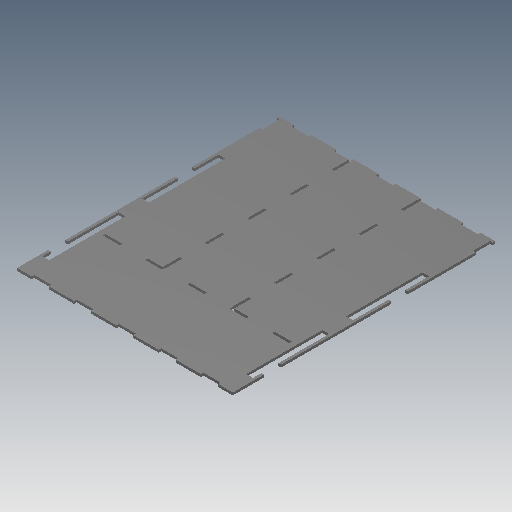
# Autodesk Inventor part: base
Saved by Autodesk Inventor 2020 (Build 240168000, 168)
## iProperties
Created: 2021-09-21
Part Number: base
Material: Generic
Document SubType Name: Modeling
Designer: pablo
Density: 1 g/cm^3
Appearance: Smooth - Black
Mass: 365.55 g
Surface Area: 1587.23 cm^2
Volume: 365.55 cm^3
Author: pablo
Autodesk Inventor part; units mm, degrees
ref_plane "YZ Plane" through (0, 0, 0) normal (1, 0, 0) x (0, 1, 0)
ref_plane "XZ Plane" through (0, 0, 0) normal (0, 1, 0) x (-1, 0, 0)
ref_plane "XY Plane" through (0, 0, 0) normal (0, 0, 1) x (1, 0, 0)
sketch "Sketch1" plane through (0, 0, 0) normal (0, 1, 0) x (-1, 0, 0)
  line L0 (127.5, -155) -> (-127.5, -155)
  line L1 (-127.5, -155) -> (-127.5, 155)
  line L2 (-127.5, 155) -> (127.5, 155)
  line L3 (127.5, 155) -> (127.5, -155)
  line L4 (127.5, -155) -> (-127.5, 155) construction
  line L5 (-127.5, -155) -> (127.5, 155) construction
  point P0 (0, 0)
  dimension "d0" = 255
  dimension "d1" = 310
  constraints: 12 end point, 2 midpoint, 2 parallel, 1 horizontal, 1 perpendicular
  measures "d0" distance of L1.end L2.end
  measures "d1" distance of L0.end L1.end
extrude "base" add sketch "Sketch1" along normal blind 3
sketch "Sketch4" plane through (0, 3, 0) normal (0, 1, 0) x (1, 0, 0)
  line L0 (-42.333, 152) -> (-39.333, 152)
  line L1 (-39.333, 152) -> (-39.333, 132)
  line L2 (-39.333, 132) -> (-42.333, 132)
  line L3 (-42.333, 132) -> (-42.333, 152)
  line L4 (39.3337, 152) -> (42.3337, 152)
  line L5 (42.3337, 152) -> (42.3337, 132)
  line L6 (42.3337, 132) -> (39.3337, 132)
  line L7 (39.3337, 132) -> (39.3337, 152)
  line L8 (-42.333, 102) -> (-39.333, 102)
  line L9 (-39.333, 102) -> (-39.333, 82)
  line L10 (-39.333, 82) -> (-42.333, 82)
  line L11 (-42.333, 82) -> (-42.333, 102)
  line L12 (39.3337, 102) -> (42.3337, 102)
  line L13 (42.3337, 102) -> (42.3337, 82)
  line L14 (42.3337, 82) -> (39.3337, 82)
  line L15 (39.3337, 82) -> (39.3337, 102)
  line L16 (-42.333, 52) -> (-39.333, 52)
  line L17 (-39.333, 52) -> (-39.333, 32)
  line L18 (-39.333, 32) -> (-42.333, 32)
  line L19 (-42.333, 32) -> (-42.333, 52)
  line L20 (39.3337, 52) -> (42.3337, 52)
  line L21 (42.3337, 52) -> (42.3337, 32)
  line L22 (42.3337, 32) -> (39.3337, 32)
  line L23 (39.3337, 32) -> (39.3337, 52)
  line L24 (-42.333, 2) -> (-39.333, 2)
  line L25 (-39.333, 2) -> (-39.333, -18)
  line L26 (-39.333, -18) -> (-42.333, -18)
  line L27 (-42.333, -18) -> (-42.333, 2)
  line L28 (39.3337, 2) -> (42.3337, 2)
  line L29 (42.3337, 2) -> (42.3337, -18)
  line L30 (42.3337, -18) -> (39.3337, -18)
  line L31 (39.3337, -18) -> (39.3337, 2)
  line L32 (-42.333, -48) -> (-39.333, -48)
  line L33 (-39.333, -48) -> (-39.333, -68)
  line L34 (-39.333, -68) -> (-42.333, -68)
  line L35 (-42.333, -68) -> (-42.333, -48)
  line L36 (39.3337, -48) -> (42.3337, -48)
  line L37 (42.3337, -48) -> (42.3337, -68)
  line L38 (42.3337, -68) -> (39.3337, -68)
  line L39 (39.3337, -68) -> (39.3337, -48)
  line L40 (0, 2.9944) -> (0, 16.9632)
  line L41 (127.5, 155) -> (-127.5, 155) projected
  point P0 (0, 0)
  dimension "d23" = 3
  dimension "d24" = 20
  dimension "d28" = 81.6667
  dimension "d31" = 50
  dimension "d93" = 39.333
  dimension "d94" = 39.3337
  dimension "d95" = 3
  constraints: 82 end point, 2 collinear, 2 horizontal, 2 parallel, 2 vertical, 1 perpendicular, 70 other
  measures "d23" distance of L1.end L2.end
  measures "d24" distance of L0.end L1.end
  measures "d28" distance of L0.start L4.start
  measures "d31" distance of L0.start L8.start
  measures "d93" horizontal distance of point (0, 0) L1.end
  measures "d94" horizontal distance of L6.end point (0, 0)
  measures "d95" distance from line of L41 L0.start
extrude "Encaixe Central" cut sketch "Sketch4" against normal blind 5
sketch "Sketch5" plane through (0, 3, 0) normal (0, 1, 0) x (1, 0, 0)
  line L0 (-127.5, -155) -> (127.5, -155) projected
  line L1 (-110, -155) -> (-90, -155)
  line L2 (-90, -155) -> (-90, -152)
  line L3 (-90, -152) -> (-110, -152)
  line L4 (-110, -152) -> (-110, -155)
  line L5 (-60, -155) -> (-40, -155)
  line L6 (-40, -155) -> (-40, -152)
  line L7 (-40, -152) -> (-60, -152)
  line L8 (-60, -152) -> (-60, -155)
  line L9 (-10, -155) -> (10, -155)
  line L10 (10, -155) -> (10, -152)
  line L11 (10, -152) -> (-10, -152)
  line L12 (-10, -152) -> (-10, -155)
  line L13 (40, -155) -> (60, -155)
  line L14 (60, -155) -> (60, -152)
  line L15 (60, -152) -> (40, -152)
  line L16 (40, -152) -> (40, -155)
  line L17 (90, -155) -> (110, -155)
  line L18 (110, -155) -> (110, -152)
  line L19 (110, -152) -> (90, -152)
  line L20 (90, -152) -> (90, -155)
  line L21 (-110, 155) -> (-110, 152)
  line L22 (-90, 155) -> (-110, 155)
  line L23 (-110, 152) -> (-90, 152)
  line L24 (-90, 152) -> (-90, 155)
  line L25 (-60, 155) -> (-60, 152)
  line L26 (-40, 155) -> (-60, 155)
  line L27 (-40, 152) -> (-40, 155)
  line L28 (-10, 155) -> (-10, 152)
  line L29 (10, 155) -> (-10, 155)
  line L30 (10, 152) -> (10, 155)
  line L31 (-10, 152) -> (10, 152)
  line L32 (-60, 152) -> (-40, 152)
  line L33 (40, 155) -> (40, 152)
  line L34 (40, 152) -> (60, 152)
  line L35 (60, 155) -> (40, 155)
  line L36 (60, 152) -> (60, 155)
  line L37 (90, 155) -> (90, 152)
  line L38 (90, 152) -> (110, 152)
  line L39 (110, 155) -> (90, 155)
  line L40 (110, 152) -> (110, 155)
  point P0 (0, 0)
  dimension "d36" = 20
  dimension "d37" = 3
  dimension "d40" = 50
  dimension "d45" = 17.5
  dimension "d46" = 17.5
  dimension "d49" = 307
  constraints: 80 end point, 2 horizontal, 2 parallel, 1 collinear, 1 perpendicular, 1 point on line, 1 vertical, 71 other
  measures "d36" distance of L3.end L2.end
  measures "d37" distance of L2.end L1.end
  measures "d40" distance of L1.start L5.start
  measures "d45" distance of L0.start L1.start
  measures "d46" distance of L17.end L0.end
  measures "d49" distance of L1.start L21.end
extrude "Encaixes frontais" cut sketch "Sketch5" against normal blind 5
sketch "Sketch6" plane through (0, 3, 0) normal (0, 1, 0) x (1, 0, 0)
  line L0 (-110, -155) -> (-110, -152) projected
  line L1 (110, -152) -> (110, -155) projected
  line L2 (-39.333, -68) -> (-42.333, -68) projected
  line L3 (-110, -68) -> (-90, -68)
  line L4 (-90, -68) -> (-90, -71)
  line L5 (-90, -71) -> (-110, -71)
  line L6 (-110, -71) -> (-110, -68)
  line L7 (-60, -68) -> (-40, -68)
  line L8 (-40, -68) -> (-40, -71)
  line L9 (-40, -71) -> (-60, -71)
  line L10 (-60, -71) -> (-60, -68)
  line L11 (-10, -68) -> (10, -68)
  line L12 (10, -68) -> (10, -71)
  line L13 (10, -71) -> (-10, -71)
  line L14 (-10, -71) -> (-10, -68)
  line L15 (40, -68) -> (60, -68)
  line L16 (60, -68) -> (60, -71)
  line L17 (60, -71) -> (40, -71)
  line L18 (40, -71) -> (40, -68)
  line L19 (90, -68) -> (110, -68)
  line L20 (110, -68) -> (110, -71)
  line L21 (110, -71) -> (90, -71)
  line L22 (90, -71) -> (90, -68)
  line L23 (-110, 155) -> (-127.5, 155) projected
  line L24 (-127.5, 155) -> (-127.5, -155) projected
  line L25 (127.5, -155) -> (127.5, 155) projected
  point P0 (0, 0)
  point P1 (-40, -68)
  dimension "d56" = 20
  dimension "d57" = 3
  dimension "d60" = 50
  dimension "d96" = 223
  dimension "d97" = 17.5
  dimension "d98" = 17.5
  constraints: 40 end point, 2 horizontal, 2 parallel, 1 collinear, 1 perpendicular, 31 other
  measures "d56" distance of L4.end L5.end
  measures "d57" distance of L3.end L4.end
  measures "d60" distance of L3.start L7.start
  measures "d96" distance from line of L23 L3.start
  measures "d97" distance from line of L24 L5.end
  measures "d98" distance from line of L25 L20.end
extrude "Encaixe longitudinal" cut sketch "Sketch6" against normal blind 5
sketch "Sketch7" plane through (0, 3, 0) normal (0, 1, 0) x (1, 0, 0)
  line L0 (-127.5, -155) -> (-110, -155) projected
  line L1 (-90, -155) -> (-60, -155) projected
  line L2 (-116.5, -10) -> (-124.5, -10)
  line L3 (-124.5, -10) -> (-124.5, 80)
  line L4 (-124.5, 80) -> (-116.5, 80)
  line L5 (-116.5, 80) -> (-116.5, -10)
  line L6 (-116.5, -10) -> (-124.5, 80) construction
  line L7 (-124.5, -10) -> (-116.5, 80) construction
  line L8 (-127.5, 155) -> (-127.5, -155) projected
  line L9 (-124.5, -128) -> (-116.5, -128)
  line L10 (-116.5, -128) -> (-116.5, -38)
  line L11 (-116.5, -38) -> (-124.5, -38)
  line L12 (-124.5, -38) -> (-124.5, -128)
  line L13 (-124.5, -128) -> (-116.5, -38) construction
  line L14 (-116.5, -128) -> (-124.5, -38) construction
  line L15 (0, -20) -> (0, -40)
  line L16 (116.5, -10) -> (124.5, -10)
  line L17 (124.5, -10) -> (124.5, 80)
  line L18 (124.5, 80) -> (116.5, 80)
  line L19 (116.5, 80) -> (116.5, -10)
  line L20 (116.5, -10) -> (124.5, 80) construction
  line L21 (124.5, -10) -> (116.5, 80) construction
  line L22 (127.5, -20) -> (127.5, -50)
  line L23 (124.5, -128) -> (116.5, -128)
  line L24 (116.5, -128) -> (116.5, -38)
  line L25 (116.5, -38) -> (124.5, -38)
  line L26 (124.5, -38) -> (124.5, -128)
  line L27 (124.5, -128) -> (116.5, -38) construction
  line L28 (116.5, -128) -> (124.5, -38) construction
  point P0 (0, 0)
  point P1 (-120.5, 35)
  point P2 (-127.5, -20)
  point P3 (-127.5, -50)
  point P4 (-120.5, -83)
  point P5 (120.5, 35)
  point P6 (120.5, -83)
  point P7 (-127.5, 150)
  dimension "d67" = 8
  dimension "d68" = 90
  dimension "d69" = 3
  dimension "d71" = 8
  dimension "d72" = 90
  dimension "d78" = 3
  dimension "d79" = 27
  dimension "d80" = 145
  constraints: 52 end point, 12 symmetric about line, 8 midpoint, 4 parallel, 2 horizontal, 2 perpendicular, 1 vertical
  measures "d67" distance of L3.end L4.end
  measures "d68" distance of L2.end L3.end
  measures "d69" distance from line of L8 L2.end
  measures "d71" distance of L11.end L10.end
  measures "d72" distance of L10.end L9.end
  measures "d78" horizontal distance of L0.start L9.start
  measures "d79" vertical distance of L0.start L9.start
  measures "d80" vertical distance of L0.start L2.end
extrude "Trajeto dos cursores" cut sketch "Sketch7" against normal blind 5
sketch "Sketch8" plane through (0, 3, 0) normal (0, 1, 0) x (1, 0, 0)
  line L0 (-127.5, 155) -> (-127.5, -155) projected
  line L1 (-110, 155) -> (-127.5, 155) projected
  line L2 (-127.5, 152) -> (-124.5, 152)
  line L3 (-124.5, 152) -> (-124.5, 132)
  line L4 (-124.5, 132) -> (-127.5, 132)
  line L5 (-127.5, 132) -> (-127.5, 152)
  line L6 (-90, 152) -> (-110, 152) projected
  line L7 (-42.333, 152) -> (-60, 152) projected
  line L8 (-127.5, 102) -> (-124.5, 102)
  line L9 (-124.5, 102) -> (-124.5, 82)
  line L10 (-124.5, 82) -> (-127.5, 82)
  line L11 (-127.5, 82) -> (-127.5, 102)
  line L12 (-127.5, 52) -> (-124.5, 52)
  line L13 (-124.5, 52) -> (-124.5, 32)
  line L14 (-124.5, 32) -> (-127.5, 32)
  line L15 (-127.5, 32) -> (-127.5, 52)
  line L16 (-127.5, 2) -> (-124.5, 2)
  line L17 (-124.5, 2) -> (-124.5, -18)
  line L18 (-124.5, -18) -> (-127.5, -18)
  line L19 (-127.5, -18) -> (-127.5, 2)
  line L20 (-127.5, -48) -> (-124.5, -48)
  line L21 (-124.5, -48) -> (-124.5, -68)
  line L22 (-124.5, -68) -> (-127.5, -68)
  line L23 (-127.5, -68) -> (-127.5, -48)
  line L24 (-127.5, -98) -> (-124.5, -98)
  line L25 (-124.5, -98) -> (-124.5, -118)
  line L26 (-124.5, -118) -> (-127.5, -118)
  line L27 (-127.5, -118) -> (-127.5, -98)
  line L28 (0, 0) -> (0, 17.1399)
  line L29 (127.5, 152) -> (124.5, 152)
  line L30 (124.5, 152) -> (124.5, 132)
  line L31 (124.5, 132) -> (127.5, 132)
  line L32 (127.5, 132) -> (127.5, 152)
  line L33 (127.5, 102) -> (124.5, 102)
  line L34 (124.5, 102) -> (124.5, 82)
  line L35 (124.5, 82) -> (127.5, 82)
  line L36 (127.5, 82) -> (127.5, 102)
  line L37 (127.5, 52) -> (124.5, 52)
  line L38 (124.5, 52) -> (124.5, 32)
  line L39 (124.5, 32) -> (127.5, 32)
  line L40 (127.5, 32) -> (127.5, 52)
  line L41 (127.5, 2) -> (124.5, 2)
  line L42 (124.5, 2) -> (124.5, -18)
  line L43 (124.5, -18) -> (127.5, -18)
  line L44 (127.5, -18) -> (127.5, 2)
  line L45 (127.5, -48) -> (124.5, -48)
  line L46 (124.5, -48) -> (124.5, -68)
  line L47 (124.5, -68) -> (127.5, -68)
  line L48 (127.5, -68) -> (127.5, -48)
  line L49 (127.5, -98) -> (124.5, -98)
  line L50 (124.5, -98) -> (124.5, -118)
  line L51 (124.5, -118) -> (127.5, -118)
  line L52 (127.5, -118) -> (127.5, -98)
  point P0 (127.5, 155)
  dimension "d82" = 3
  dimension "d83" = 20
  dimension "d86" = 50
  constraints: 98 end point, 25 symmetric about line, 2 parallel, 2 vertical, 1 horizontal, 1 perpendicular, 1 point on line, 40 other
  measures "d82" distance of L3.end L4.end
  measures "d83" distance of L2.end L3.end
  measures "d86" distance of L2.start L8.start
extrude "Encaixes latereis" cut sketch "Sketch8" against normal blind 3 contours L2 L3 L4 L0 | L12 L13 L14 L0 | L24 L25 L26 L0 | L32 L31 L30 L29 | L40 L39 L38 L37 | L52 L51 L50 L49
body "Solid1"
